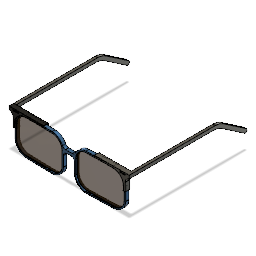
23-Day 17 - Sunglasses v1 (Autodesk Fusion 360 design; units mm, degrees)
Autodesk Fusion 360 part; units mm, degrees
sketch "Sketch1" plane through (0, 0, 0) normal (0, 0, 1) x (1, 0, 0)
  line L0 (-10, 35) -> (-10, 15)
  line L1 (10, 35) -> (10, 15)
  line L2 (-80, 35) -> (-80, 15)
  line L3 (80, 35) -> (80, 15)
  line L4 (65, 50) -> (25, 50)
  line L5 (-25, 50) -> (-65, 50)
  line L6 (-65, 0) -> (-25, 0)
  line L7 (25, 0) -> (65, 0)
  arc A0 (-65, 50) -> (-80, 35) centre (-65, 35) ccw
  arc A1 (-10, 35) -> (-25, 50) centre (-25, 35) ccw
  arc A2 (-80, 15) -> (-65, 0) centre (-65, 15) ccw
  arc A3 (-25, 0) -> (-10, 15) centre (-25, 15) ccw
  arc A4 (10, 15) -> (25, 0) centre (25, 15) ccw
  arc A5 (25, 50) -> (10, 35) centre (25, 35) ccw
  arc A6 (80, 35) -> (65, 50) centre (65, 35) ccw
  arc A7 (65, 0) -> (80, 15) centre (65, 15) ccw
  line L8 (-82, 35) -> (-82, 15)
  arc A8 (-82, 15) -> (-65, -2) centre (-65, 15) ccw
  line L9 (-65, -2) -> (-25, -2)
  arc A9 (-25, -2) -> (-8, 15) centre (-25, 15) ccw
  line L10 (-8, 30) -> (-8, 15)
  arc A10 (-9.5135, 42.012) -> (-25, 52) centre (-25, 35) ccw
  line L11 (-25, 52) -> (-65, 52)
  arc A11 (-65, 52) -> (-82, 35) centre (-65, 35) ccw
  arc A12 (8, 15) -> (25, -2) centre (25, 15) ccw
  line L12 (25, -2) -> (65, -2)
  arc A13 (65, -2) -> (82, 15) centre (65, 15) ccw
  line L13 (82, 35) -> (82, 15)
  arc A14 (82, 35) -> (65, 52) centre (65, 35) ccw
  line L14 (65, 52) -> (25, 52)
  arc A15 (25, 52) -> (9.5135, 42.012) centre (25, 35) ccw
  line L15 (8, 30) -> (8, 15)
  line L16 (-4.9587, 39.0744) -> (4.9587, 39.0744)
  line L17 (-3.3291, 35) -> (-3, 35)
  line L18 (-3.3291, 35) -> (3, 35)
  arc A16 (-9.5135, 42.012) -> (-4.9587, 39.0744) centre (-4.9587, 44.0744) ccw
  arc A17 (4.9587, 39.0744) -> (9.5135, 42.012) centre (4.9587, 44.0744) ccw
  arc A18 (-3, 35) -> (-8, 30) centre (-3, 30) ccw
  arc A19 (8, 30) -> (3, 35) centre (3, 30) ccw
  dimension "d1" = 15
  dimension "d4" = 5
  constraint horizontal L6
  constraint horizontal L4
  constraint perpendicular L0 L6
  constraint perpendicular L1 L6
  constraint perpendicular L2 L6
  constraint perpendicular L3 L6
  constraint collinear L4 L5
  constraint collinear L6 L7
  constraint tangent L2 A0
  constraint tangent L5 A0
  constraint tangent L0 A1
  constraint tangent L5 A1
  constraint equal A0 A1
  constraint tangent L2 A2
  constraint tangent L6 A2
  constraint equal A0 A2
  constraint tangent L0 A3
  constraint tangent L6 A3
  constraint equal A0 A3
  constraint tangent L1 A4
  constraint tangent L7 A4
  constraint equal A0 A4
  constraint tangent L1 A5
  constraint tangent L4 A5
  constraint equal A0 A5
  constraint tangent L3 A6
  constraint tangent L4 A6
  constraint equal A0 A6
  constraint tangent L3 A7
  constraint tangent L7 A7
  constraint equal A0 A7
  constraint perpendicular L1 L16
  constraint perpendicular L10 L17
  constraint perpendicular L15 L18
  constraint parallel L2 L8
  constraint concentric A2 A8
  constraint parallel L6 L9
  constraint concentric A3 A9
  constraint parallel L0 L10
  constraint concentric A1 A10
  constraint parallel L5 L11
  constraint concentric A0 A11
  constraint tangent L8 A11
  constraint tangent A9 L10
  constraint tangent L8 A8
  constraint tangent L9 A9
  constraint tangent A8 L9
  constraint tangent L10 A10
  constraint tangent A10 L11
  constraint tangent L11 A11
  constraint tangent L16 A16
  constraint tangent A10 A16
  constraint concentric A4 A12
  constraint parallel L7 L12
  constraint concentric A7 A13
  constraint parallel L3 L13
  constraint concentric A6 A14
  constraint parallel L4 L14
  constraint concentric A5 A15
  constraint parallel L1 L15
  constraint tangent L14 A15
  constraint tangent A14 L14
  constraint tangent A12 L15
  constraint tangent A15 L15
  constraint tangent L12 A13
  constraint tangent A12 L12
  constraint tangent A13 L13
  constraint tangent L13 A14
  constraint tangent L16 A17
  constraint tangent A15 A17
  constraint equal A16 A17
  constraint tangent L10 A18
  constraint tangent L17 A18
  constraint equal A16 A18
  constraint tangent L15 A19
  constraint tangent L18 A19
  constraint equal A16 A19
  measures "d1" radius of A0
  measures "d4" radius of A16
extrude "Extrude1" add sketch "Sketch1" against normal blind 30 makes body 1
sketch "Sketch2" plane through (0, 0, 0) normal (0, 1, 0) x (1, 0, 0)
  spline S0 degree 5 poles (-100, 10) (-96, 9.7725) (-88, 9.3372) (-76, 8.744) (-60, 8.0743) (-40, 7.4528) (-20, 7.0663) (0, 6.934) (20, 7.0663) (40, 7.4528) (60, 8.0743) (76, 8.744) (88, 9.3372) (96, 9.7725) (100, 10) knots 0 0 0 0 0 0 0.1 0.2 0.3 0.4 0.5 0.6 0.7 0.8 0.9 1 1 1 1 1 1
  spline S1 degree 3 poles (-99.716, 14.9919) (-63.2723, 12.9188) (-26.845, 11.8023) (9.5708, 12.03) (39.6059, 12.2177) (69.6579, 13.282) (99.716, 14.9919) knots 0 0 0 0 0.54801 0.54801 0.54801 1 1 1 1
  line L0 (100, 10) -> (99.716, 14.9919)
  line L1 (-100, 10) -> (-99.716, 14.9919)
  point P0 (0, 7)
  dimension "d7" = -5
extrude "Extrude2" cut sketch "Sketch2" along normal blind 60 and the other way blind 10 keep common part bodies 1
sketch "Sketch3" plane through (0, 0, 0) normal (0, 0, 1) x (1, 0, 0)
  spline S0 degree 3 poles (82, 35) (82, 35.525) (81.9757, 36.0506) (81.7188, 38.8115) (81.0695, 40.9843) (78.9813, 44.9201) (77.5749, 46.6512) (74.324, 49.3579) (72.5526, 50.3636) (69.6079, 51.4006) (68.536, 51.6646) (66.6361, 51.9409) (65.8186, 52) (65, 52) knots 4.731585 4.731585 4.731585 4.731585 4.889609 4.889609 5.563446 5.563446 6.226558 6.226558 6.833236 6.833236 7.163885 7.163885 7.409644 7.409644 7.409644 7.409644
  line L0 (65, 52) -> (25, 52)
  line L1 (82, 15) -> (82, 35)
  spline S1 degree 3 poles (65, 50) (65.6519, 50) (66.3033, 49.9575) (67.8916, 49.7493) (68.8195, 49.5366) (71.4081, 48.6783) (72.9824, 47.8234) (75.7067, 45.644) (76.8503, 44.3542) (78.7087, 41.3541) (79.3772, 39.6477) (79.9081, 36.9177) (80, 35.9588) (80, 35) knots 2.913501 2.913501 2.913501 2.913501 3.109274 3.109274 3.394441 3.394441 3.928042 3.928042 4.441657 4.441657 4.987054 4.987054 5.276047 5.276047 5.276047 5.276047
  line L2 (80, 35) -> (80, 15)
  line L3 (25, 50) -> (65, 50)
  line L4 (83, 15) -> (83, 35)
  spline S2 degree 3 poles (83, 35) (83, 35.5559) (82.9743, 36.1124) (82.9226, 36.6677) (82.7022, 39.0357) (82.0148, 41.3364) (80.9004, 43.4367) (79.8037, 45.5036) (78.3146, 47.3366) (76.517, 48.8332) (74.8724, 50.2024) (72.9969, 51.2674) (70.9788, 51.978) (69.8789, 52.3654) (68.744, 52.6449) (67.59, 52.8127) (66.7323, 52.9374) (65.8667, 53) (65, 53) knots 4.731585 4.731585 4.731585 4.731585 4.889609 4.889609 4.889609 5.563446 5.563446 5.563446 6.226558 6.226558 6.226558 6.833236 6.833236 6.833236 7.163885 7.163885 7.163885 7.409644 7.409644 7.409644 7.409644
  line L5 (65, 53) -> (25, 53)
  line L6 (25, 49) -> (65, 49)
  spline S3 degree 3 poles (65, 49) (65.6085, 49) (66.2164, 48.9603) (66.8198, 48.8812) (67.6988, 48.766) (68.5649, 48.5675) (69.4063, 48.2885) (70.9809, 47.7664) (72.4503, 46.9685) (73.7458, 45.9321) (74.9929, 44.9344) (76.0602, 43.7306) (76.9015, 42.3726) (77.7948, 40.9305) (78.4187, 39.3379) (78.7426, 37.6724) (78.9142, 36.7899) (79, 35.8949) (79, 35) knots 2.913501 2.913501 2.913501 2.913501 3.109274 3.109274 3.109274 3.394441 3.394441 3.394441 3.928042 3.928042 3.928042 4.441657 4.441657 4.441657 4.987054 4.987054 4.987054 5.276047 5.276047 5.276047 5.276047
  line L7 (79, 35) -> (79, 15)
  line L8 (65, 53) -> (83, 53)
  line L9 (83, 35) -> (83, 53)
  line L10 (37.4824, 49) -> (37.4824, 53)
  line L11 (79, 28.5337) -> (83, 28.5337)
  line L12 (83, 53) -> (90, 53)
  line L13 (90, 53) -> (90, 47.9987)
  line L14 (90, 47.9987) -> (83, 47.9987)
  dimension "d12" = 1
  dimension "d13" = 1
  constraint parallel L0 L8
  constraint coincident L6 L10.start
  constraint coincident L5 L10.end
  constraint perpendicular L5 L10
  constraint coincident L7 L11.start
  constraint coincident L4 L11.end
  constraint perpendicular L4 L11
  constraint perpendicular L9 L12
  constraint perpendicular L12 L13
  constraint coincident L9 L14.end
  constraint perpendicular L9 L14
extrude "Extrude3" add sketch "Sketch3" against normal blind 7 from surface at -7.3 separate body makes body 2
fillet "Fillet1" radius 1.5 6 edges at (79, 31.7668, -14.3) (74.9019, 44.8971, -14.3) (51.2412, 49, -14.3) (51.2412, 49, -7.3) (74.9019, 44.8971, -7.3) (79, 31.7668, -7.3) on bodies 2
fillet "Fillet3" radius 7 1 edges at (83, 47.9987, -10.8) on bodies 2
extrude "Extrude4" cut 2 faces at (89.9995, 47.9987, -9.6333) (90, 51.3329, -9.6333) along direction (-1, 0, 0) blind 1 on bodies 2 bodies 2
extrude "Extrude5" cut 1 faces at (89.6653, 47.9987, -9.6333) along direction (0, -1, 0) blind 2 on bodies 2 bodies 2
sketch "Sketch4" plane through (0, 0, -7.3) normal (0, 0, 1) x (1, 0, 0)
  line L0 (89, 47.9269) -> (89, 53)
  line L1 (89, 53) -> (37.4824, 53)
  line L2 (37.4824, 53) -> (37.4824, 50.5)
  line L3 (37.4824, 50.5) -> (65, 50.5)
  spline S0 degree 3 poles (80.5, 35) (80.5, 35.9906) (80.4042, 36.9859) (80.215, 37.9587) (79.8584, 39.7923) (79.1689, 41.5607) (77.5288, 44.2083) (76.7533, 45.1783) (75.5198, 46.3951) (75.1344, 46.7393) (73.2157, 48.2871) (71.4706, 49.2186) (68.1228, 50.2621) (66.55, 50.5) (65, 50.5) knots 0 0 0 0 0.297174 0.297174 0.297174 0.857309 0.857309 1.22304 1.22304 1.377116 1.377116 1.957262 1.957262 2.422261 2.422261 2.422261 2.422261
  line L4 (80.5, 35) -> (80.5, 28.5337)
  line L5 (80.5, 28.5337) -> (83, 28.5337)
  line L6 (83, 28.5337) -> (83, 40.9987)
  arc A0 (89, 47.9269) -> (83, 40.9987) centre (90, 40.9987) ccw
  line L7 (83, 50) -> (75, 50)
  line L8 (75, 50) -> (75, 51)
  line L9 (75, 51) -> (83, 51)
  line L10 (83, 51) -> (83, 50)
  constraint horizontal L7
  constraint vertical L8
  constraint horizontal L9
  constraint vertical L10
extrude "Extrude6" cut sketch "Sketch4" against normal blind 0.5 contours L7 L8 L9 L10 bodies 2
mirror "Mirror1" about plane through (0, 0, 0) normal (1, 0, 0) of bodies 2 makes body 3
sketch "Sketch5" plane through (89, 0, 0) normal (1, 0, 0) x (0, 0, -1)
  line L0 (7.3, 53) -> (7.3, 47.9269)
  line L1 (7.3, 47.9269) -> (14.3, 47.9269)
  line L2 (14.3, 47.9269) -> (14.3, 53)
  line L3 (14.3, 53) -> (7.3, 53)
  line L4 (14.3, 53) -> (134.6158, 53)
  line L5 (132.1974, 47.996) -> (14.3, 47.9269)
  line L6 (144.6174, 44.1637) -> (177.9355, 21.4099)
  line L7 (181.4099, 22.0645) -> (181.6856, 22.4683)
  line L8 (181.031, 25.9427) -> (147.0229, 49.1676)
  arc A0 (144.6174, 44.1637) -> (132.1974, 47.996) centre (132.2103, 25.996) ccw
  arc A1 (147.0229, 49.1676) -> (134.6158, 53) centre (134.6158, 31) ccw
  arc A2 (177.9355, 21.4099) -> (181.4099, 22.0645) centre (179.3454, 23.4744) ccw
  arc A3 (181.6856, 22.4683) -> (181.031, 25.9427) centre (179.6211, 23.8782) ccw
  dimension "d37" = 22
  dimension "d38" = 2.5
  constraint coincident L2.end L3.start
  constraint perpendicular L2 L4
  constraint coincident L1.end L2.start
  constraint perpendicular L6 L7
  constraint perpendicular L7 L8
  constraint tangent L5 A0
  constraint tangent L6 A0
  constraint tangent L8 A1
  constraint tangent L4 A1
  constraint equal A0 A1
  constraint tangent L6 A2
  constraint tangent L7 A2
  constraint tangent L7 A3
  constraint tangent L8 A3
  constraint equal A2 A3
  measures "d37" radius of A0
  measures "d38" radius of A2
extrude "Extrude7" add sketch "Sketch5" against normal blind 4 contours L2 L4 L5 L6 L7 L8 A0 A1 A2 A3 bodies 2
mirror "Mirror2" about plane through (0, 0, 0) normal (1, 0, 0) of "Extrude7" makes body 4
extrude "Extrude8" add sketch "Sketch1" along normal blind 1 from surface at -10 separate body contours L0 L2 L5 L6 A0 A1 A2 A3 | L1 L3 L4 L7 A4 A5 A6 A7 makes body 5 at (51.6667, 33.3333, -10) makes body 6 at (-51.6667, 33.3333, -10)
